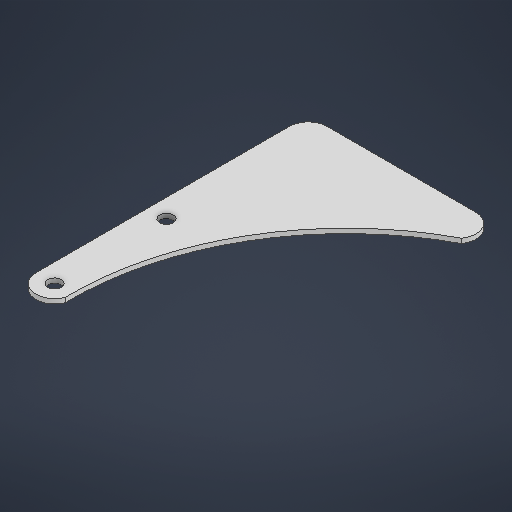
# Autodesk Inventor part: Lady Brown Tabs
Saved by Autodesk Inventor 2025 (Build 290162000, 162)
## iProperties
Created: 2024-12-29
Part Number: Lady Brown Tabs
Material: Generic
Document SubType Name: Modeling
Designer: Juan
Density: 1 g/cm^3
Appearance: Default
Author: Juan
Autodesk Inventor part; units mm, degrees
ref_plane "YZ Plane" through (0, 0, 0) normal (1, 0, 0) x (0, 1, 0)
ref_plane "XZ Plane" through (0, 0, 0) normal (0, 1, 0) x (-1, 0, 0)
ref_plane "XY Plane" through (0, 0, 0) normal (0, 0, 1) x (1, 0, 0)
sketch "Sketch1" plane through (0, 0, 0) normal (0, 1, 0) x (-1, 0, 0)
  circle A0 centre (0, 0) radius 2.3241
  line L0 (0, 0) -> (0, -38.1)
  circle A1 centre (0, -38.1) radius 2.3241
  line L1 (0, 0) -> (0, -38.1) construction
  line L2 (-6.35, 0) -> (-6.35, -38.1)
  line L3 (6.35, -38.1) -> (6.35, 0)
  arc A2 (6.35, 0) -> (-6.35, 0) centre (0, 0) ccw
  arc A3 (-6.35, -38.1) -> (6.35, -38.1) centre (0, -38.1) ccw
  line L4 (0, -38.1) -> (-15.9411, -38.1) construction
  line L5 (0, -31.75) -> (-15.9411, -31.75)
  line L6 (-15.9411, -44.45) -> (0, -44.45)
  arc A4 (0, -44.45) -> (0, -31.75) centre (0, -38.1) ccw
  arc A5 (-15.9411, -31.75) -> (-15.9411, -44.45) centre (-15.9411, -38.1) ccw
  line L7 (-5.9094, 2.3241) -> (-21.799, -35.6488)
  point P0 (0, -19.05)
  point P1 (-7.9706, -38.1)
  dimension "d0" = 4.6482
  dimension "d1" = 38.1
  dimension "d2" = 4.6482
  dimension "d3" = 12.7
  constraints: 20 end point, 10 point on circle, 9 tangent, 6 centre point, 3 equal length, 2 coincident, 2 midpoint, 1 perpendicular, 1 vertical
  measures "d0" diameter of A0
  measures "d1" distance of L0.start L0.end
  measures "d2" diameter of A1
  measures "d3" diameter of A3
extrude "Extrusion1" add sketch "Sketch1" along normal blind 1.5875
sketch "Sketch2" plane through (0, 1.5875, 0) normal (0, 1, 0) x (1, 0, 0)
  circle A0 centre (0, 38.1) radius 2.3241 projected
  line L0 (0, 38.1) -> (0, 31.75)
  line L1 (0, 31.75) -> (0, 92.71) construction
  line L2 (6.35, 38.1) -> (6.35, 86.36)
  line L3 (-6.35, 86.36) -> (-6.35, 38.1)
  arc A1 (-6.35, 38.1) -> (6.35, 38.1) centre (0, 38.1) ccw
  arc A2 (6.35, 86.36) -> (-6.35, 86.36) centre (0, 86.36) ccw
  line L4 (-6.35, 86.36) -> (57.15, 86.36) construction
  line L5 (0, 80.01) -> (50.8, 80.01)
  line L6 (50.8, 92.71) -> (0, 92.71)
  arc A3 (0, 92.71) -> (0, 80.01) centre (0, 86.36) ccw
  arc A4 (50.8, 80.01) -> (50.8, 92.71) centre (50.8, 86.36) ccw
  line L7 (-6.35, 38.1) -> (-6.35, 0) projected
  arc A5 (-6.35, 0) -> (5.9094, -2.3241) centre (0, 0) ccw projected
  line L8 (5.9094, -2.3241) -> (21.799, 35.6488) projected
  arc A6 (21.799, 35.6488) -> (15.9411, 44.45) centre (15.9411, 38.1) ccw projected
  line L9 (15.9411, 44.45) -> (0, 44.45) projected
  arc A7 (0, 44.45) -> (-6.35, 38.1) centre (0, 38.1) ccw projected
  circle A8 centre (0, 0) radius 2.3241 projected
  circle A9 centre (0, 38.1) radius 2.3241 projected
  line L10 (21.799, 35.6488) -> (55.9369, 82.6271)
  point P0 (0, 62.23)
  point P1 (25.4, 86.36)
  point P2 (0, 92.71)
  point P3 (6.35, 44.45)
  dimension "d6" = 6.35
  dimension "d7" = 60.96
  dimension "d10" = 63.5
  constraints: 20 end point, 13 point on circle, 9 tangent, 4 centre point, 4 point on line, 2 midpoint, 2 parallel, 2 vertical, 1 horizontal
  measures "d6" distance of L0.start L0.end
  measures "d7" distance of L0.end L1.end
  measures "d10" distance of L3.start L4.end
extrude "Extrusion2" add sketch "Sketch2" against normal blind 1.5875 contours A1 A7 L9 L2 | L9 A7 L3 A3 L5 L2 | L2 L5 A4 L10 A6 L9 | L5 A3 A2 L2 | L2 A2 L6 A4 L5
sketch "Sketch3" plane through (0, 1.5875, 0) normal (0, 1, 0) x (1, 0, 0)
  arc A0 (55.9369, 82.6271) -> (50.8, 92.71) centre (50.8, 86.36) ccw projected
  line L0 (5.9094, -2.3241) -> (21.799, 35.6488) projected
  arc A1 (55.9369, 82.6271) -> (5.9094, -2.3241) centre (99.8414, -0.4343) ccw
  line L1 (21.799, 35.6488) -> (55.9369, 82.6271) projected
  point P0 (0, 0)
  constraints: 2 point on circle, 1 centre point
extrude "Extrusion3" cut sketch "Sketch3" against normal blind 1.5875
body "Solid1"
